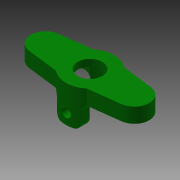
# Autodesk Inventor part: ServoHornPocket2
Saved by Autodesk Inventor 2014 SP1 (Build 180222100, 222)
## iProperties
Created: 2017-01-17
Part Number: ServoHornPocket2
Material: Generic
Document SubType Name: Modeling
Designer: danielsikar
Density: 1 g/cm^3
Appearance: Dark Green
Author: danielsikar
Autodesk Inventor part; units mm, degrees
ref_plane "YZ Plane" through (0, 0, 0) normal (1, 0, 0) x (0, 1, 0)
ref_plane "XZ Plane" through (0, 0, 0) normal (0, 1, 0) x (-1, 0, 0)
ref_plane "XY Plane" through (0, 0, 0) normal (0, 0, 1) x (1, 0, 0)
sketch "bASE" plane through (0, 0, 0) normal (0, 0, 1) x (1, 0, 0)
  arc A0 (-16.7865, 2.679) -> (-16.7865, -2.679) centre (-16.45, 0) ccw
  arc A1 (16.7865, -2.679) -> (16.7865, 2.679) centre (16.45, 0) ccw
  line L0 (4.4678, -4.2262) -> (16.7865, -2.679)
  line L1 (4.4678, 4.2262) -> (16.7865, 2.679)
  line L2 (-4.4678, 4.2262) -> (-16.7865, 2.679)
  line L3 (-4.4678, -4.2262) -> (-16.7865, -2.679)
  arc A2 (-4.4678, -4.2262) -> (4.4678, -4.2262) centre (0, 0) ccw
  arc A3 (4.4678, 4.2262) -> (-4.4678, 4.2262) centre (0, 0) ccw
  point P0 (0, 4.2262)
  dimension "d20" = 5.4
  dimension "d21" = 5.4
  constraints: 8 end point, 8 point on circle, 4 centre point, 4 tangent, 1 coincident, 1 vertical alignment
  measures "d20" diameter of A0
  measures "d21" diameter of A1
sketch "Coupling" plane through (0, 0, 0) normal (0, 0, 1) x (1, 0, 0)
  line L0 (-4.4678, 4.2262) -> (-16.7865, 2.679) projected
  arc A0 (4.4678, 4.2262) -> (-4.4678, 4.2262) centre (0, 0) ccw projected
  line L1 (4.4678, 4.2262) -> (16.7865, 2.679) projected
  arc A1 (16.7865, -2.679) -> (16.7865, 2.679) centre (16.45, 0) ccw projected
  line L2 (4.4678, -4.2262) -> (16.7865, -2.679) projected
  arc A2 (-4.4678, -4.2262) -> (4.4678, -4.2262) centre (0, 0) ccw projected
  line L3 (-4.4678, -4.2262) -> (-16.7865, -2.679) projected
  arc A3 (-16.7865, 2.679) -> (-16.7865, -2.679) centre (-16.45, 0) ccw projected
  line L4 (17.1339, 5.4452) -> (5.7046, 6.8807)
  arc A4 (5.7046, 6.8807) -> (-5.7046, 6.8807) centre (0, 0) ccw
  line L5 (-5.7046, 6.8807) -> (-17.1339, 5.4452)
  arc A5 (-17.1339, 5.4452) -> (-17.1339, -5.4452) centre (-16.45, 0) ccw
  line L6 (-17.1339, -5.4452) -> (-5.7046, -6.8807)
  arc A6 (-5.7046, -6.8807) -> (5.7046, -6.8807) centre (0, 0) ccw
  line L7 (5.7046, -6.8807) -> (17.1339, -5.4452)
  arc A7 (17.1339, -5.4452) -> (17.1339, 5.4452) centre (16.45, 0) ccw
  constraints: 8 end point, 8 point on circle, 4 centre point, 7 other
extrude "Extrusion7" add sketch "Coupling" along normal blind 5.5 contours A0 L1 A1 L2 A2 L3 A3 L0 | A7 L7 A6 L6 A5 L5 A4 L4
extrude "Extrusion8" cut sketch "bASE" along normal blind 3
sketch "Sketch8" plane through (0, 0, 3) normal (0, 0, -1) x (-1, 0, 0)
  arc A0 (-4.4678, -4.2262) -> (4.4678, -4.2262) centre (0, 0) ccw projected
  circle A1 centre (0, 0) radius 4.55
  dimension "d26" = 9.1
  constraints: 1 centre point, 1 coincident
  measures "d26" diameter of A1
extrude "Extrusion9" cut sketch "Sketch8" against normal blind 3
sketch "Sketch9" plane through (0, 0, 0) normal (0, 0, -1) x (-1, 0, 0)
  arc A0 (4.4678, 4.2262) -> (-4.4678, 4.2262) centre (0, 0) ccw projected
  line L0 (4.4678, 4.2262) -> (16.7865, 2.679) projected
  arc A1 (16.7865, -2.679) -> (16.7865, 2.679) centre (16.45, 0) ccw projected
  line L1 (16.7865, -2.679) -> (4.4678, -4.2262) projected
  arc A2 (-4.4678, -4.2262) -> (4.4678, -4.2262) centre (0, 0) ccw projected
  line L2 (-4.4678, -4.2262) -> (-16.7865, -2.679) projected
  arc A3 (-16.7865, 2.679) -> (-16.7865, -2.679) centre (-16.45, 0) ccw projected
  line L3 (-16.7865, 2.679) -> (-4.4678, 4.2262) projected
  line L4 (16.8276, 3.0059) -> (4.6244, 4.5387)
  arc A4 (4.6244, 4.5387) -> (-4.6244, 4.5387) centre (0, 0) ccw
  line L5 (-4.6244, 4.5387) -> (-16.8276, 3.0059)
  arc A5 (-16.8276, 3.0059) -> (-16.8276, -3.0059) centre (-16.45, 0) ccw
  line L6 (-16.8276, -3.0059) -> (-4.6244, -4.5387)
  arc A6 (-4.6244, -4.5387) -> (4.6244, -4.5387) centre (0, 0) ccw
  line L7 (4.6244, -4.5387) -> (16.8276, -3.0059)
  arc A7 (16.8276, -3.0059) -> (16.8276, 3.0059) centre (16.45, 0) ccw
  constraints: 8 end point, 8 point on circle, 4 centre point, 7 other
extrude "Extrusion10" cut sketch "Sketch9" against normal up to surface (3 mm away)
sketch "Sketch10" plane through (0, 0, 0) normal (0, 0, -1) x (-1, 0, 0)
  arc A0 (-4.6244, -4.5387) -> (4.6244, -4.5387) centre (0, 0) ccw projected
  line L0 (-4.6244, -4.5387) -> (-16.8276, -3.0059) projected
  line L1 (-16.8276, 3.0059) -> (-4.6244, 4.5387) projected
  arc A1 (4.6244, 4.5387) -> (-4.6244, 4.5387) centre (0, 0) ccw projected
  line L2 (4.6244, 4.5387) -> (16.8276, 3.0059) projected
  line L3 (16.8276, -3.0059) -> (4.6244, -4.5387) projected
  arc A2 (-5.7046, -6.8807) -> (5.7046, -6.8807) centre (0, 0) ccw projected
  arc A3 (5.7046, 6.8807) -> (-5.7046, 6.8807) centre (0, 0) ccw projected
  arc A4 (-4.6244, -4.5387) -> (4.6244, -4.5387) centre (0, 0) ccw
  arc A5 (4.6244, 4.5387) -> (-4.6244, 4.5387) centre (0, 0) ccw
  line L4 (4.5, 7.7225) -> (4.5, 4.662)
  line L5 (4.5, -4.662) -> (4.5, -7.7225)
  line L6 (-4.5, -7.7225) -> (-4.5, -4.662)
  line L7 (-4.5, 4.662) -> (-4.5, 7.7225)
  point P0 (4.5, 0)
  constraints: 12 end point, 12 point on circle, 4 parallel, 2 centre point, 1 coincident
extrude "Extrusion11" add sketch "Sketch10" along normal blind 8
sketch "Sketch11" plane through (0, 0, 0) normal (0, 1, 0) x (-1, 0, 0)
  arc A0 (-8.5, -3.2) -> (-11.5, -3.2) centre (-10, -4) ccw projected
  spline S0 degree 3 poles (-11.7, -4) (-11.7, -4.2199) (-11.655, -4.4494) (-11.4803, -4.8659) (-11.3506, -5.0536) (-11.0543, -5.3499) (-10.8664, -5.4801) (-10.4488, -5.6552) (-10.2188, -5.7) (-9.7812, -5.7) (-9.5512, -5.6552) (-9.1336, -5.4801) (-8.9457, -5.3499) (-8.6494, -5.0536) (-8.5197, -4.8659) (-8.345, -4.4494) (-8.3, -4.2199) (-8.3, -3.7801) (-8.345, -3.5506) (-8.5197, -3.1341) (-8.6494, -2.9464) (-8.9457, -2.6501) (-9.1336, -2.5199) (-9.5512, -2.3448) (-9.7812, -2.3) (-10.2188, -2.3) (-10.4488, -2.3448) (-10.8664, -2.5199) (-11.0543, -2.6501) (-11.3506, -2.9464) (-11.4803, -3.1341) (-11.655, -3.5506) (-11.7, -3.7801) (-11.7, -4) knots 0 0 0 0 0.065958 0.065958 0.131917 0.131917 0.197553 0.197553 0.263189 0.263189 0.328824 0.328824 0.39446 0.39446 0.460419 0.460419 0.526377 0.526377 0.592335 0.592335 0.658294 0.658294 0.72393 0.72393 0.789566 0.789566 0.855201 0.855201 0.920837 0.920837 0.986796 0.986796 1.052754 1.052754 1.052754 1.052754 projected
  point P0 (0, 0)
  point P1 (-11.7, -4)
extrude "Extrusion12" cut sketch "Sketch11" along normal through all both and the other way through all
fillet "Fillet1" radius 2 8 edges at (-4.5, 6.1923, 0) (-4.5, -6.1923, 0) (4.5, 6.1923, 0) (4.5, -6.1923, 0) (4.5, -6.1923, -8) (4.5, 6.1923, -8) (-4.5, 6.1923, -8) (-4.5, -6.1923, -8)
body "Solid3"
